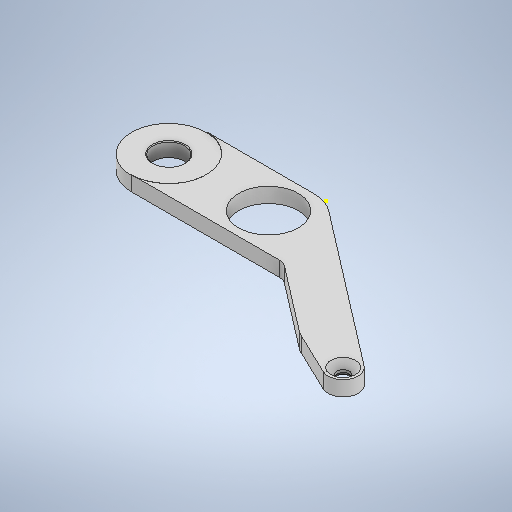
# Autodesk Inventor part: 31-10-201-novi
Saved by Autodesk Inventor 2025.2 (Build 292293000, 293)
## iProperties
Created: 2024-11-28
Part Number: 31-10-201-novi
Material: Generic
Document SubType Name: Modeling
Designer: Zvonko.Gabric
Density: 1 g/cm^3
Appearance: Default
Description: Tension lever, Belt tensioner
Author: Zvonko.Gabric
Autodesk Inventor part; units mm, degrees
ref_plane "YZ Plane" through (0, 0, 0) normal (1, 0, 0) x (0, 1, 0)
ref_plane "XZ Plane" through (0, 0, 0) normal (0, 1, 0) x (-1, 0, 0)
sketch "Sketch1" plane through (0, 0, 0) normal (0, 1, 0) x (-1, 0, 0)
  line L0 (0, 0) -> (48.2762, -0.0067)
  line L1 (-64.893, 49.805) -> (0, 0)
  line L2 (-40.6563, 51.3726) -> (-58.6663, 59.989)
  line L3 (-12.8113, 30.0018) -> (-40.6563, 51.3726)
  line L4 (48.2788, 29.9933) -> (-12.8113, 30.0018)
  arc A0 (-58.6663, 59.989) -> (-64.893, 49.805) centre (-61.2549, 54.5762) ccw
  arc A1 (48.2762, -0.0067) -> (48.2788, 29.9933) centre (48.2762, 14.9933) ccw
  point P0 (0, 0)
  dimension "d0" = 0
  dimension "d1" = 0
  dimension "d2" = 15
  dimension "d3" = 48.2762
  dimension "d4" = 48.2762
  dimension "d5" = 61.0901
  dimension "d6" = 109.5311
  dimension "d7" = 6
  dimension "d8" = 168.062
  dimension "d9" = 30
  dimension "d10" = 16
  dimension "d11" = 18.01
  constraints: 10 end point, 4 point on circle, 2 centre point
  measures "d0" distance of point (0, 0) L0.start
  measures "d1" distance of point (0, 0) L0.start
  measures "d2" radius of A1
  measures "d3" horizontal distance of point (0, 0) A1.centre
  measures "d4" distance of L0.start L0.end
  measures "d5" distance of L4.start L3.start
  measures "d6" horizontal distance of A0.centre A1.centre
  measures "d7" radius of A0
  measures "d8" angle of L2 L3
  measures "d9" distance between parallel lines of L0 L4
  measures "d10" distance between parallel lines of L3 L1
  measures "d11" horizontal distance of L2.start L2.end
extrude "Extrusion1" add sketch "Sketch1" along normal blind 6
sketch "Sketch2" plane through (0, 6, 0) normal (0, 1, 0) x (1, 0, 0)
  arc A0 (-48.2762, 0.0067) -> (-48.2788, -29.9933) centre (-48.2762, -14.9933) ccw projected
  circle A1 centre (-48.2762, -14.9933) radius 15
  point P0 (0, 0)
  point P1 (-48.2788, -29.9933)
  point P2 (-48.2762, 0.0067)
  constraints: 1 centre point, 1 coincident
extrude "Extrusion2" cut sketch "Sketch2" against normal blind 0.3
sketch "Sketch3" plane through (0, 6, 0) normal (0, 1, 0) x (1, 0, 0)
  circle A0 centre (-8.2762, -14.9988) radius 12
  arc A1 (-48.2762, 0.0067) -> (-48.2788, -29.9933) centre (-48.2762, -14.9933) ccw projected
  line L0 (-48.2788, -29.9933) -> (12.8113, -30.0018) projected
  point P0 (0, 0)
  point P1 (-63.2762, -14.992)
  dimension "d16" = 55
  dimension "d17" = 15
  dimension "d18" = 24
  constraints: 1 centre point, 1 point on circle
  measures "d16" distance of point (-63.276, -14.992) A0.centre
  measures "d17" distance from line of L0 A0.centre
  measures "d18" diameter of A0
extrude "Extrusion3" cut sketch "Sketch3" against normal blind 10
sketch "Sketch8" plane through (0, 5.7, 0) normal (0, 1, 0) x (1, 0, 0)
  arc A0 (-48.2762, 0.0067) -> (-48.2788, -29.9933) centre (-48.2762, -14.9933) ccw projected
  circle A1 centre (-48.2762, -14.9933) radius 6.3
  point P0 (0, 0)
  dimension "d37" = 12.6
  constraints: 1 centre point, 1 coincident
  measures "d37" diameter of A1
extrude "Extrusion4" cut sketch "Sketch8" against normal blind 10
chamfer "Chamfer1" distance 0.3 angle 45 1 edges at (-54.5762, 5.7, 14.9933) measured on face at (-46.8281, 5.7, 26.9329)
fillet "Fillet1" radius 15 1 edges at (0, 3, 0)
fillet "Fillet2" radius 5 1 edges at (12.8113, 3, 30.0018)
fillet "Fillet3" radius 10 1 edges at (40.6563, 3, 51.3726)
sketch "Sketch15" plane through (64.893, 0, 49.805) normal (0.6088, 0, -0.7933) x (-0.7933, 0, -0.6088)
  point P0 (81.8024, 0)
sketch "Sketch16" plane through (0, 6, 0) normal (0, 1, 0) x (1, 0, 0)
  point P0 (0, 0)
ref_plane "Work Plane3" through (61.2399, 0, 54.5647) normal (0.6088, 0, -0.7933) x (-0.7933, 0, -0.6088)
sketch "Sketch18" plane through (61.2399, 0, 54.5647) normal (0.6088, 0, -0.7933) x (-0.7933, 0, -0.6088)
  line L0 (0, 6) -> (76.7109, 6) projected
  line L1 (0, 6) -> (0, 3.5)
  line L2 (0, 0) -> (0, 6) projected
  line L3 (-2.5, 3.5) -> (-5, 6)
  line L4 (0, 6) -> (-6.0189, 6) projected
  line L5 (-2.5, 3.5) -> (0, 3.5)
  line L6 (-6.0189, 0) -> (-6.0189, 6) projected
  line L7 (-6.0189, 3) -> (0, 3) construction
  line L8 (0, 0) -> (0, 2.5)
  line L9 (-2.5, 2.5) -> (-5, 0)
  line L10 (-2.5, 2.5) -> (0, 2.5)
  line L11 (-5, 0) -> (0, 0)
  line L12 (17.2493, 0) -> (-1.2609, 0) projected
  point P0 (81.8024, 0)
  point P1 (-1.2609, 6)
  point P2 (0, 2.5)
  dimension "d75" = 2.5
  dimension "d76" = 2.5
  dimension "d77" = 5
  constraints: 16 end point, 3 symmetric about line, 2 midpoint, 2 point on line, 1 collinear, 1 perpendicular
  measures "d75" horizontal distance of L3.start L3.end
  measures "d76" distance from line of L1 L3.start
  measures "d77" distance from line of L1 L3.end
revolve "Revolution1" cut sketch "Sketch18" angle 360 about axis through (61.2399, 6, 54.5647) along (0, -1, 0)
sketch "Sketch19" plane through (61.2399, 3.5, 54.5647) normal (0, 1, 0) x (1, 0, 0)
  circle A0 centre (0, 0) radius 2.5
  point P0 (-61.2399, 54.5647)
  constraints: 1 centre point
extrude "Extrusion6" cut sketch "Sketch19" against normal blind 10
body "Solid1"
